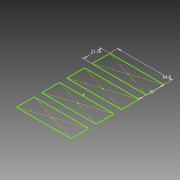
# Autodesk Inventor part: UNLHEP-14-01-P-006_SensorMock
Saved by Autodesk Inventor 2013 (Build 170138000, 138)
## iProperties
Created: 2014-01-06
Part Number: UNLHEP-14-01-P-006_SensorMock
Material: Allgemein
Document SubType Name: Modeling
Designer: Frank Meier
Density: 1 g/cm^3
Project: UNL Pixel Phase I
Author: Frank Meier
Revision Number: 00
Autodesk Inventor part; units mm, degrees
ref_plane "YZ Plane" through (0, 0, 0) normal (1, 0, 0) x (0, 1, 0)
ref_plane "XZ Plane" through (0, 0, 0) normal (0, 1, 0) x (-1, 0, 0)
ref_plane "XY Plane" through (0, 0, 0) normal (0, 0, 1) x (1, 0, 0)
sketch "Skizze1" plane through (0, 0, 0) normal (0, 0, 1) x (1, 0, 0)
  line L0 (37.5144, 58.2287) -> (-27.2856, 58.2287)
  line L1 (-27.2856, 58.2287) -> (-27.2856, 37.0687)
  line L2 (-27.2856, 37.0687) -> (37.5144, 37.0687)
  line L3 (37.5144, 37.0687) -> (37.5144, 58.2287)
  line L4 (37.5144, 58.2287) -> (-27.2856, 37.0687) construction
  line L5 (-27.2856, 58.2287) -> (37.5144, 37.0687) construction
  line L6 (37.5144, 28.2287) -> (-27.2856, 28.2287)
  line L7 (-27.2856, 28.2287) -> (-27.2856, 7.0687)
  line L8 (-27.2856, 7.0687) -> (37.5144, 7.0687)
  line L9 (37.5144, 7.0687) -> (37.5144, 28.2287)
  line L10 (37.5144, 28.2287) -> (-27.2856, 7.0687) construction
  line L11 (-27.2856, 28.2287) -> (37.5144, 7.0687) construction
  line L12 (37.5144, -1.7713) -> (-27.2856, -1.7713)
  line L13 (-27.2856, -1.7713) -> (-27.2856, -22.9313)
  line L14 (-27.2856, -22.9313) -> (37.5144, -22.9313)
  line L15 (37.5144, -22.9313) -> (37.5144, -1.7713)
  line L16 (37.5144, -1.7713) -> (-27.2856, -22.9313) construction
  line L17 (-27.2856, -1.7713) -> (37.5144, -22.9313) construction
  line L18 (37.5144, -31.7713) -> (-27.2856, -31.7713)
  line L19 (-27.2856, -31.7713) -> (-27.2856, -52.9313)
  line L20 (-27.2856, -52.9313) -> (37.5144, -52.9313)
  line L21 (37.5144, -52.9313) -> (37.5144, -31.7713)
  line L22 (37.5144, -31.7713) -> (-27.2856, -52.9313) construction
  line L23 (-27.2856, -31.7713) -> (37.5144, -52.9313) construction
  point P0 (0, 0)
  point P1 (5.1144, 47.6487)
  point P2 (5.1144, 17.6487)
  point P3 (5.1144, -12.3513)
  point P4 (5.1144, -42.3513)
  dimension "d0" = 64.8
  dimension "d2" = 21.16
  dimension "d5" = 30
  constraints: 48 end point, 8 midpoint, 2 parallel, 1 collinear, 1 horizontal, 1 perpendicular, 1 vertical, 32 other
  measures "d0" distance between parallel lines of L3 L1
  measures "d2" distance of L0.end L1.end
  measures "d5" distance of L0.start L6.start
extrude "Extrusion1" add sketch "Skizze1" along normal blind 0.17
